Autodesk Inventor part; units mm, degrees
(part 2 of 2)
sketch "Sketch6" plane through (0, 0, 150.495) normal (1, 0, 0) x (0, 0, -1)
  arc A0 (27.7241, 58.674) -> (29.8831, 58.674) centre (28.8036, 58.674) ccw
  line L0 (29.8831, 83.82) -> (29.8831, 58.674)
  line L1 (27.7241, 83.82) -> (27.7241, 58.674)
  line L2 (28.8036, 59.7535) -> (28.8036, 58.674)
  line L3 (28.8036, 83.82) -> (28.8036, 82.7405)
  arc A1 (29.8831, 83.82) -> (27.7241, 83.82) centre (28.8036, 83.82) ccw
  line L4 (28.8036, 55.626) -> (28.8036, 54.5465)
  arc A2 (29.8831, 55.626) -> (27.7241, 55.626) centre (28.8036, 55.626) ccw
  line L5 (27.7241, 55.626) -> (27.7241, 30.48)
  line L6 (29.8831, 55.626) -> (29.8831, 30.48)
  arc A3 (27.7241, 30.48) -> (29.8831, 30.48) centre (28.8036, 30.48) ccw
  line L7 (28.8036, 31.5595) -> (28.8036, 30.48)
  line L8 (28.8036, 27.432) -> (28.8036, 26.3525)
  arc A4 (29.8831, 27.432) -> (27.7241, 27.432) centre (28.8036, 27.432) ccw
  line L9 (29.8831, 27.432) -> (29.8831, 2.286)
  line L10 (27.7241, 27.432) -> (27.7241, 2.286)
  line L11 (28.8036, 3.3655) -> (28.8036, 2.286)
  arc A5 (27.7241, 2.286) -> (29.8831, 2.286) centre (28.8036, 2.286) ccw
  arc A6 (31.8643, 58.674) -> (34.0233, 58.674) centre (32.9438, 58.674) ccw
  line L12 (32.9438, 59.7535) -> (32.9438, 58.674)
  arc A7 (36.0045, 58.674) -> (38.1635, 58.674) centre (37.084, 58.674) ccw
  line L13 (31.8643, 83.82) -> (31.8643, 58.674)
  line L14 (38.1635, 83.82) -> (38.1635, 58.674)
  line L15 (34.0233, 83.82) -> (34.0233, 58.674)
  line L16 (36.0045, 83.82) -> (36.0045, 58.674)
  line L17 (37.084, 59.7535) -> (37.084, 58.674)
  line L18 (32.9438, 83.82) -> (32.9438, 81.8268)
  arc A8 (34.0233, 83.82) -> (31.8643, 83.82) centre (32.9438, 83.82) ccw
  line L19 (37.084, 83.82) -> (37.084, 82.7405)
  arc A9 (38.1635, 83.82) -> (36.0045, 83.82) centre (37.084, 83.82) ccw
  line L20 (32.9438, 55.626) -> (32.9438, 53.2839)
  arc A10 (34.0233, 55.626) -> (31.8643, 55.626) centre (32.9438, 55.626) ccw
  line L21 (37.084, 55.626) -> (37.084, 54.5465)
  arc A11 (38.1635, 55.626) -> (36.0045, 55.626) centre (37.084, 55.626) ccw
  line L22 (31.8643, 55.626) -> (31.8643, 30.48)
  line L23 (32.9438, 31.5595) -> (32.9438, 30.48)
  line L24 (36.0045, 55.626) -> (36.0045, 30.48)
  line L25 (38.1635, 55.626) -> (38.1635, 30.48)
  line L26 (34.0233, 55.626) -> (34.0233, 30.48)
  arc A12 (31.8643, 30.48) -> (34.0233, 30.48) centre (32.9438, 30.48) ccw
  arc A13 (36.0045, 30.48) -> (38.1635, 30.48) centre (37.084, 30.48) ccw
  line L27 (37.084, 31.5595) -> (37.084, 30.48)
  arc A14 (34.0233, 27.432) -> (31.8643, 27.432) centre (32.9438, 27.432) ccw
  line L28 (37.084, 27.432) -> (37.084, 26.3525)
  arc A15 (38.1635, 27.432) -> (36.0045, 27.432) centre (37.084, 27.432) ccw
  line L29 (32.9438, 27.432) -> (32.9438, 26.3525)
  line L30 (38.1635, 27.432) -> (38.1635, 2.286)
  line L31 (36.0045, 27.432) -> (36.0045, 2.286)
  line L32 (34.0233, 27.432) -> (34.0233, 2.286)
  line L33 (31.8643, 27.432) -> (31.8643, 2.286)
  line L34 (37.084, 3.3655) -> (37.084, 2.286)
  line L35 (32.9438, 3.3655) -> (32.9438, 2.286)
  arc A16 (36.0045, 2.286) -> (38.1635, 2.286) centre (37.084, 2.286) ccw
  arc A17 (31.8643, 2.286) -> (34.0233, 2.286) centre (32.9438, 2.286) ccw
  arc A18 (40.1447, 58.674) -> (42.3037, 58.674) centre (41.2242, 58.674) ccw
  line L36 (41.2242, 59.7535) -> (41.2242, 58.674)
  arc A19 (44.2849, 58.674) -> (46.4439, 58.674) centre (45.3644, 58.674) ccw
  line L37 (40.1447, 83.82) -> (40.1447, 58.674)
  line L38 (46.4439, 83.82) -> (46.4439, 58.674)
  line L39 (42.3037, 83.82) -> (42.3037, 58.674)
  line L40 (44.2849, 83.82) -> (44.2849, 58.674)
  line L41 (45.3644, 59.7535) -> (45.3644, 58.674)
  line L42 (41.2242, 83.82) -> (41.2242, 81.8268)
  arc A20 (42.3037, 83.82) -> (40.1447, 83.82) centre (41.2242, 83.82) ccw
  line L43 (45.3644, 83.82) -> (45.3644, 82.7405)
  arc A21 (46.4439, 83.82) -> (44.2849, 83.82) centre (45.3644, 83.82) ccw
  line L44 (41.2242, 55.626) -> (41.2242, 53.2839)
  arc A22 (42.3037, 55.626) -> (40.1447, 55.626) centre (41.2242, 55.626) ccw
  line L45 (45.3644, 55.626) -> (45.3644, 54.5465)
  arc A23 (46.4439, 55.626) -> (44.2849, 55.626) centre (45.3644, 55.626) ccw
  line L46 (40.1447, 55.626) -> (40.1447, 30.48)
  line L47 (41.2242, 31.5595) -> (41.2242, 30.48)
  line L48 (44.2849, 55.626) -> (44.2849, 30.48)
  line L49 (46.4439, 55.626) -> (46.4439, 30.48)
  line L50 (42.3037, 55.626) -> (42.3037, 30.48)
  arc A24 (40.1447, 30.48) -> (42.3037, 30.48) centre (41.2242, 30.48) ccw
  arc A25 (44.2849, 30.48) -> (46.4439, 30.48) centre (45.3644, 30.48) ccw
  line L51 (45.3644, 31.5595) -> (45.3644, 30.48)
  arc A26 (42.3037, 27.432) -> (40.1447, 27.432) centre (41.2242, 27.432) ccw
  line L52 (45.3644, 27.432) -> (45.3644, 26.3525)
  arc A27 (46.4439, 27.432) -> (44.2849, 27.432) centre (45.3644, 27.432) ccw
  line L53 (41.2242, 27.432) -> (41.2242, 26.3525)
  line L54 (46.4439, 27.432) -> (46.4439, 2.286)
  line L55 (44.2849, 27.432) -> (44.2849, 2.286)
  line L56 (42.3037, 27.432) -> (42.3037, 2.286)
  line L57 (40.1447, 27.432) -> (40.1447, 2.286)
  line L58 (45.3644, 3.3655) -> (45.3644, 2.286)
  line L59 (41.2242, 3.3655) -> (41.2242, 2.286)
  arc A28 (44.2849, 2.286) -> (46.4439, 2.286) centre (45.3644, 2.286) ccw
  arc A29 (40.1447, 2.286) -> (42.3037, 2.286) centre (41.2242, 2.286) ccw
  arc A30 (50.5841, 83.82) -> (48.4251, 83.82) centre (49.5046, 83.82) ccw
  line L60 (49.5046, 83.82) -> (49.5046, 81.8268)
  line L61 (53.6448, 83.82) -> (53.6448, 82.7405)
  arc A31 (54.7243, 83.82) -> (52.5653, 83.82) centre (53.6448, 83.82) ccw
  line L62 (48.4251, 83.82) -> (48.4251, 58.674)
  line L63 (49.5046, 59.7535) -> (49.5046, 58.674)
  line L64 (50.5841, 83.82) -> (50.5841, 58.674)
  line L65 (52.5653, 83.82) -> (52.5653, 58.674)
  line L66 (54.7243, 83.82) -> (54.7243, 58.674)
  line L67 (53.6448, 55.626) -> (53.6448, 54.5465)
  line L68 (49.5046, 55.626) -> (49.5046, 53.2839)
  line L69 (54.7243, 55.626) -> (54.7243, 30.48)
  line L70 (53.6448, 31.5595) -> (53.6448, 30.48)
  line L71 (52.5653, 55.626) -> (52.5653, 30.48)
  line L72 (50.5841, 55.626) -> (50.5841, 30.48)
  line L73 (49.5046, 31.5595) -> (49.5046, 30.48)
  line L74 (48.4251, 55.626) -> (48.4251, 30.48)
  arc A32 (50.5841, 55.626) -> (48.4251, 55.626) centre (49.5046, 55.626) ccw
  arc A33 (54.7243, 55.626) -> (52.5653, 55.626) centre (53.6448, 55.626) ccw
  arc A34 (48.4251, 58.674) -> (50.5841, 58.674) centre (49.5046, 58.674) ccw
  arc A35 (52.5653, 58.674) -> (54.7243, 58.674) centre (53.6448, 58.674) ccw
  line L75 (53.6448, 59.7535) -> (53.6448, 58.674)
  arc A36 (52.5653, 30.48) -> (54.7243, 30.48) centre (53.6448, 30.48) ccw
  arc A37 (48.4251, 30.48) -> (50.5841, 30.48) centre (49.5046, 30.48) ccw
  arc A38 (54.7243, 27.432) -> (52.5653, 27.432) centre (53.6448, 27.432) ccw
  arc A39 (50.5841, 27.432) -> (48.4251, 27.432) centre (49.5046, 27.432) ccw
  line L76 (49.5046, 27.432) -> (49.5046, 26.3525)
  line L77 (53.6448, 27.432) -> (53.6448, 26.3525)
  line L78 (54.7243, 27.432) -> (54.7243, 2.286)
  line L79 (52.5653, 27.432) -> (52.5653, 2.286)
  line L80 (50.5841, 27.432) -> (50.5841, 2.286)
  line L81 (48.4251, 27.432) -> (48.4251, 2.286)
  line L82 (53.6448, 3.3655) -> (53.6448, 2.286)
  line L83 (49.5046, 3.3655) -> (49.5046, 2.286)
  arc A40 (52.5653, 2.286) -> (54.7243, 2.286) centre (53.6448, 2.286) ccw
  arc A41 (48.4251, 2.286) -> (50.5841, 2.286) centre (49.5046, 2.286) ccw
  arc A42 (58.8645, 83.82) -> (56.7055, 83.82) centre (57.785, 83.82) ccw
  line L84 (57.785, 83.82) -> (57.785, 81.8268)
  line L85 (61.9252, 83.82) -> (61.9252, 82.7405)
  arc A43 (63.0047, 83.82) -> (60.8457, 83.82) centre (61.9252, 83.82) ccw
  line L86 (56.7055, 83.82) -> (56.7055, 58.674)
  line L87 (57.785, 59.7535) -> (57.785, 58.674)
  line L88 (58.8645, 83.82) -> (58.8645, 58.674)
  line L89 (60.8457, 83.82) -> (60.8457, 58.674)
  line L90 (63.0047, 83.82) -> (63.0047, 58.674)
  line L91 (61.9252, 55.626) -> (61.9252, 54.5465)
  line L92 (57.785, 55.626) -> (57.785, 53.2839)
  line L93 (63.0047, 55.626) -> (63.0047, 30.48)
  line L94 (61.9252, 31.5595) -> (61.9252, 30.48)
  line L95 (60.8457, 55.626) -> (60.8457, 30.48)
  line L96 (58.8645, 55.626) -> (58.8645, 30.48)
  line L97 (57.785, 31.5595) -> (57.785, 30.48)
  line L98 (56.7055, 55.626) -> (56.7055, 30.48)
  arc A44 (58.8645, 55.626) -> (56.7055, 55.626) centre (57.785, 55.626) ccw
  arc A45 (63.0047, 55.626) -> (60.8457, 55.626) centre (61.9252, 55.626) ccw
  arc A46 (56.7055, 58.674) -> (58.8645, 58.674) centre (57.785, 58.674) ccw
  arc A47 (60.8457, 58.674) -> (63.0047, 58.674) centre (61.9252, 58.674) ccw
  line L99 (61.9252, 59.7535) -> (61.9252, 58.674)
  arc A48 (60.8457, 30.48) -> (63.0047, 30.48) centre (61.9252, 30.48) ccw
  arc A49 (56.7055, 30.48) -> (58.8645, 30.48) centre (57.785, 30.48) ccw
  arc A50 (63.0047, 27.432) -> (60.8457, 27.432) centre (61.9252, 27.432) ccw
  arc A51 (58.8645, 27.432) -> (56.7055, 27.432) centre (57.785, 27.432) ccw
  line L100 (57.785, 27.432) -> (57.785, 26.3525)
  line L101 (61.9252, 27.432) -> (61.9252, 26.3525)
  line L102 (63.0047, 27.432) -> (63.0047, 2.286)
  line L103 (60.8457, 27.432) -> (60.8457, 2.286)
  line L104 (58.8645, 27.432) -> (58.8645, 2.286)
  line L105 (56.7055, 27.432) -> (56.7055, 2.286)
  line L106 (61.9252, 3.3655) -> (61.9252, 2.286)
  line L107 (57.785, 3.3655) -> (57.785, 2.286)
  arc A52 (60.8457, 2.286) -> (63.0047, 2.286) centre (61.9252, 2.286) ccw
  arc A53 (56.7055, 2.286) -> (58.8645, 2.286) centre (57.785, 2.286) ccw
  arc A54 (67.1449, 83.82) -> (64.9859, 83.82) centre (66.0654, 83.82) ccw
  line L108 (66.0654, 83.82) -> (66.0654, 81.8268)
  line L109 (70.2056, 83.82) -> (70.2056, 82.7405)
  arc A55 (71.2851, 83.82) -> (69.1261, 83.82) centre (70.2056, 83.82) ccw
  line L110 (64.9859, 83.82) -> (64.9859, 58.674)
  line L111 (66.0654, 59.7535) -> (66.0654, 58.674)
  line L112 (67.1449, 83.82) -> (67.1449, 58.674)
  line L113 (69.1261, 83.82) -> (69.1261, 58.674)
  line L114 (71.2851, 83.82) -> (71.2851, 58.674)
  line L115 (70.2056, 55.626) -> (70.2056, 54.5465)
  line L116 (66.0654, 55.626) -> (66.0654, 53.2839)
  line L117 (71.2851, 55.626) -> (71.2851, 30.48)
  line L118 (70.2056, 31.5595) -> (70.2056, 30.48)
  line L119 (69.1261, 55.626) -> (69.1261, 30.48)
  line L120 (67.1449, 55.626) -> (67.1449, 30.48)
  line L121 (66.0654, 31.5595) -> (66.0654, 30.48)
  line L122 (64.9859, 55.626) -> (64.9859, 30.48)
  arc A56 (67.1449, 55.626) -> (64.9859, 55.626) centre (66.0654, 55.626) ccw
  arc A57 (71.2851, 55.626) -> (69.1261, 55.626) centre (70.2056, 55.626) ccw
  arc A58 (64.9859, 58.674) -> (67.1449, 58.674) centre (66.0654, 58.674) ccw
  arc A59 (69.1261, 58.674) -> (71.2851, 58.674) centre (70.2056, 58.674) ccw
  line L123 (70.2056, 59.7535) -> (70.2056, 58.674)
  arc A60 (69.1261, 30.48) -> (71.2851, 30.48) centre (70.2056, 30.48) ccw
  arc A61 (64.9859, 30.48) -> (67.1449, 30.48) centre (66.0654, 30.48) ccw
  arc A62 (71.2851, 27.432) -> (69.1261, 27.432) centre (70.2056, 27.432) ccw
  arc A63 (67.1449, 27.432) -> (64.9859, 27.432) centre (66.0654, 27.432) ccw
  line L124 (66.0654, 27.432) -> (66.0654, 26.3525)
  line L125 (70.2056, 27.432) -> (70.2056, 26.3525)
  line L126 (71.2851, 27.432) -> (71.2851, 2.286)
  line L127 (69.1261, 27.432) -> (69.1261, 2.286)
  line L128 (67.1449, 27.432) -> (67.1449, 2.286)
  line L129 (64.9859, 27.432) -> (64.9859, 2.286)
  line L130 (70.2056, 3.3655) -> (70.2056, 2.286)
  line L131 (66.0654, 3.3655) -> (66.0654, 2.286)
  arc A64 (69.1261, 2.286) -> (71.2851, 2.286) centre (70.2056, 2.286) ccw
  arc A65 (64.9859, 2.286) -> (67.1449, 2.286) centre (66.0654, 2.286) ccw
  arc A66 (73.2663, 58.674) -> (75.4253, 58.674) centre (74.3458, 58.674) ccw
  line L132 (74.3458, 59.7535) -> (74.3458, 58.674)
  arc A67 (77.4065, 58.674) -> (79.5655, 58.674) centre (78.486, 58.674) ccw
  line L133 (73.2663, 83.82) -> (73.2663, 58.674)
  line L134 (79.5655, 83.82) -> (79.5655, 58.674)
  line L135 (75.4253, 83.82) -> (75.4253, 58.674)
  line L136 (77.4065, 83.82) -> (77.4065, 58.674)
  line L137 (78.486, 59.7535) -> (78.486, 58.674)
  line L138 (74.3458, 83.82) -> (74.3458, 81.8268)
  arc A68 (75.4253, 83.82) -> (73.2663, 83.82) centre (74.3458, 83.82) ccw
  line L139 (78.486, 83.82) -> (78.486, 82.7405)
  arc A69 (79.5655, 83.82) -> (77.4065, 83.82) centre (78.486, 83.82) ccw
  line L140 (74.3458, 55.626) -> (74.3458, 53.2839)
  arc A70 (75.4253, 55.626) -> (73.2663, 55.626) centre (74.3458, 55.626) ccw
  line L141 (78.486, 55.626) -> (78.486, 54.5465)
  arc A71 (79.5655, 55.626) -> (77.4065, 55.626) centre (78.486, 55.626) ccw
  line L142 (73.2663, 55.626) -> (73.2663, 30.48)
  line L143 (74.3458, 31.5595) -> (74.3458, 30.48)
  line L144 (77.4065, 55.626) -> (77.4065, 30.48)
  line L145 (79.5655, 55.626) -> (79.5655, 30.48)
  line L146 (75.4253, 55.626) -> (75.4253, 30.48)
  arc A72 (73.2663, 30.48) -> (75.4253, 30.48) centre (74.3458, 30.48) ccw
  arc A73 (77.4065, 30.48) -> (79.5655, 30.48) centre (78.486, 30.48) ccw
  line L147 (78.486, 31.5595) -> (78.486, 30.48)
  arc A74 (75.4253, 27.432) -> (73.2663, 27.432) centre (74.3458, 27.432) ccw
  line L148 (78.486, 27.432) -> (78.486, 26.3525)
  arc A75 (79.5655, 27.432) -> (77.4065, 27.432) centre (78.486, 27.432) ccw
  line L149 (74.3458, 27.432) -> (74.3458, 26.3525)
  line L150 (79.5655, 27.432) -> (79.5655, 2.286)
  line L151 (77.4065, 27.432) -> (77.4065, 2.286)
  line L152 (75.4253, 27.432) -> (75.4253, 2.286)
  line L153 (73.2663, 27.432) -> (73.2663, 2.286)
  line L154 (78.486, 3.3655) -> (78.486, 2.286)
  line L155 (74.3458, 3.3655) -> (74.3458, 2.286)
  arc A76 (77.4065, 2.286) -> (79.5655, 2.286) centre (78.486, 2.286) ccw
  arc A77 (73.2663, 2.286) -> (75.4253, 2.286) centre (74.3458, 2.286) ccw
  arc A78 (83.7057, 83.82) -> (81.5467, 83.82) centre (82.6262, 83.82) ccw
  line L156 (82.6262, 83.82) -> (82.6262, 81.8268)
  line L157 (86.7664, 83.82) -> (86.7664, 82.7405)
  arc A79 (87.8459, 83.82) -> (85.6869, 83.82) centre (86.7664, 83.82) ccw
  line L158 (81.5467, 83.82) -> (81.5467, 58.674)
  line L159 (82.6262, 59.7535) -> (82.6262, 58.674)
  line L160 (83.7057, 83.82) -> (83.7057, 58.674)
  line L161 (85.6869, 83.82) -> (85.6869, 58.674)
  line L162 (87.8459, 83.82) -> (87.8459, 58.674)
  line L163 (86.7664, 55.626) -> (86.7664, 54.5465)
  line L164 (82.6262, 55.626) -> (82.6262, 53.2839)
  line L165 (87.8459, 55.626) -> (87.8459, 30.48)
  line L166 (86.7664, 31.5595) -> (86.7664, 30.48)
  line L167 (85.6869, 55.626) -> (85.6869, 30.48)
  line L168 (83.7057, 55.626) -> (83.7057, 30.48)
  line L169 (82.6262, 31.5595) -> (82.6262, 30.48)
  line L170 (81.5467, 55.626) -> (81.5467, 30.48)
  arc A80 (83.7057, 55.626) -> (81.5467, 55.626) centre (82.6262, 55.626) ccw
  arc A81 (87.8459, 55.626) -> (85.6869, 55.626) centre (86.7664, 55.626) ccw
  arc A82 (81.5467, 58.674) -> (83.7057, 58.674) centre (82.6262, 58.674) ccw
  arc A83 (85.6869, 58.674) -> (87.8459, 58.674) centre (86.7664, 58.674) ccw
  line L171 (86.7664, 59.7535) -> (86.7664, 58.674)
  arc A84 (85.6869, 30.48) -> (87.8459, 30.48) centre (86.7664, 30.48) ccw
  arc A85 (81.5467, 30.48) -> (83.7057, 30.48) centre (82.6262, 30.48) ccw
  arc A86 (87.8459, 27.432) -> (85.6869, 27.432) centre (86.7664, 27.432) ccw
  arc A87 (83.7057, 27.432) -> (81.5467, 27.432) centre (82.6262, 27.432) ccw
  line L172 (82.6262, 27.432) -> (82.6262, 26.3525)
  line L173 (86.7664, 27.432) -> (86.7664, 26.3525)
  line L174 (87.8459, 27.432) -> (87.8459, 2.286)
  line L175 (85.6869, 27.432) -> (85.6869, 2.286)
  line L176 (83.7057, 27.432) -> (83.7057, 2.286)
  line L177 (81.5467, 27.432) -> (81.5467, 2.286)
  line L178 (86.7664, 3.3655) -> (86.7664, 2.286)
  line L179 (82.6262, 3.3655) -> (82.6262, 2.286)
  arc A88 (85.6869, 2.286) -> (87.8459, 2.286) centre (86.7664, 2.286) ccw
  arc A89 (81.5467, 2.286) -> (83.7057, 2.286) centre (82.6262, 2.286) ccw
  arc A90 (91.9861, 83.82) -> (89.8271, 83.82) centre (90.9066, 83.82) ccw
  line L180 (90.9066, 83.82) -> (90.9066, 81.8268)
  line L181 (95.0468, 83.82) -> (95.0468, 82.7405)
  arc A91 (96.1263, 83.82) -> (93.9673, 83.82) centre (95.0468, 83.82) ccw
  line L182 (89.8271, 83.82) -> (89.8271, 58.674)
  line L183 (90.9066, 59.7535) -> (90.9066, 58.674)
  line L184 (91.9861, 83.82) -> (91.9861, 58.674)
  line L185 (93.9673, 83.82) -> (93.9673, 58.674)
  line L186 (96.1263, 83.82) -> (96.1263, 58.674)
  line L187 (95.0468, 55.626) -> (95.0468, 54.5465)
  line L188 (90.9066, 55.626) -> (90.9066, 53.2839)
  line L189 (96.1263, 55.626) -> (96.1263, 30.48)
  line L190 (95.0468, 31.5595) -> (95.0468, 30.48)
  line L191 (93.9673, 55.626) -> (93.9673, 30.48)
  line L192 (91.9861, 55.626) -> (91.9861, 30.48)
  line L193 (90.9066, 31.5595) -> (90.9066, 30.48)
  line L194 (89.8271, 55.626) -> (89.8271, 30.48)
  arc A92 (91.9861, 55.626) -> (89.8271, 55.626) centre (90.9066, 55.626) ccw
  arc A93 (96.1263, 55.626) -> (93.9673, 55.626) centre (95.0468, 55.626) ccw
  arc A94 (89.8271, 58.674) -> (91.9861, 58.674) centre (90.9066, 58.674) ccw
  arc A95 (93.9673, 58.674) -> (96.1263, 58.674) centre (95.0468, 58.674) ccw
  line L195 (95.0468, 59.7535) -> (95.0468, 58.674)
  arc A96 (93.9673, 30.48) -> (96.1263, 30.48) centre (95.0468, 30.48) ccw
  arc A97 (89.8271, 30.48) -> (91.9861, 30.48) centre (90.9066, 30.48) ccw
  arc A98 (96.1263, 27.432) -> (93.9673, 27.432) centre (95.0468, 27.432) ccw
  arc A99 (91.9861, 27.432) -> (89.8271, 27.432) centre (90.9066, 27.432) ccw
  line L196 (90.9066, 27.432) -> (90.9066, 26.3525)
  line L197 (95.0468, 27.432) -> (95.0468, 26.3525)
  line L198 (96.1263, 27.432) -> (96.1263, 2.286)
  line L199 (93.9673, 27.432) -> (93.9673, 2.286)
  line L200 (91.9861, 27.432) -> (91.9861, 2.286)
  line L201 (89.8271, 27.432) -> (89.8271, 2.286)
  line L202 (95.0468, 3.3655) -> (95.0468, 2.286)
  line L203 (90.9066, 3.3655) -> (90.9066, 2.286)
  arc A100 (93.9673, 2.286) -> (96.1263, 2.286) centre (95.0468, 2.286) ccw
  arc A101 (89.8271, 2.286) -> (91.9861, 2.286) centre (90.9066, 2.286) ccw
  arc A102 (100.2665, 83.82) -> (98.1075, 83.82) centre (99.187, 83.82) ccw
  line L204 (99.187, 83.82) -> (99.187, 81.8268)
  line L205 (103.3272, 83.82) -> (103.3272, 82.7405)
  arc A103 (104.4067, 83.82) -> (102.2477, 83.82) centre (103.3272, 83.82) ccw
  line L206 (98.1075, 83.82) -> (98.1075, 58.674)
  line L207 (99.187, 59.7535) -> (99.187, 58.674)
  line L208 (100.2665, 83.82) -> (100.2665, 58.674)
  line L209 (102.2477, 83.82) -> (102.2477, 58.674)
  line L210 (104.4067, 83.82) -> (104.4067, 58.674)
  line L211 (103.3272, 55.626) -> (103.3272, 54.5465)
  line L212 (99.187, 55.626) -> (99.187, 53.2839)
  line L213 (104.4067, 55.626) -> (104.4067, 30.48)
  line L214 (103.3272, 31.5595) -> (103.3272, 30.48)
  line L215 (102.2477, 55.626) -> (102.2477, 30.48)
  line L216 (100.2665, 55.626) -> (100.2665, 30.48)
  line L217 (99.187, 31.5595) -> (99.187, 30.48)
  line L218 (98.1075, 55.626) -> (98.1075, 30.48)
  arc A104 (100.2665, 55.626) -> (98.1075, 55.626) centre (99.187, 55.626) ccw
  arc A105 (104.4067, 55.626) -> (102.2477, 55.626) centre (103.3272, 55.626) ccw
  arc A106 (98.1075, 58.674) -> (100.2665, 58.674) centre (99.187, 58.674) ccw
  arc A107 (102.2477, 58.674) -> (104.4067, 58.674) centre (103.3272, 58.674) ccw
  line L219 (103.3272, 59.7535) -> (103.3272, 58.674)
  arc A108 (102.2477, 30.48) -> (104.4067, 30.48) centre (103.3272, 30.48) ccw
  arc A109 (98.1075, 30.48) -> (100.2665, 30.48) centre (99.187, 30.48) ccw
  arc A110 (104.4067, 27.432) -> (102.2477, 27.432) centre (103.3272, 27.432) ccw
  arc A111 (100.2665, 27.432) -> (98.1075, 27.432) centre (99.187, 27.432) ccw
  line L220 (99.187, 27.432) -> (99.187, 26.3525)
  line L221 (103.3272, 27.432) -> (103.3272, 26.3525)
  line L222 (104.4067, 27.432) -> (104.4067, 2.286)
  line L223 (102.2477, 27.432) -> (102.2477, 2.286)
  line L224 (100.2665, 27.432) -> (100.2665, 2.286)
  line L225 (98.1075, 27.432) -> (98.1075, 2.286)
  line L226 (103.3272, 3.3655) -> (103.3272, 2.286)
  line L227 (99.187, 3.3655) -> (99.187, 2.286)
  arc A112 (102.2477, 2.286) -> (104.4067, 2.286) centre (103.3272, 2.286) ccw
  arc A113 (98.1075, 2.286) -> (100.2665, 2.286) centre (99.187, 2.286) ccw
  arc A114 (106.3879, 58.674) -> (108.5469, 58.674) centre (107.4674, 58.674) ccw
  arc A115 (110.5281, 58.674) -> (112.6871, 58.674) centre (111.6076, 58.674) ccw
  line L228 (111.6076, 59.7535) -> (111.6076, 58.674)
  arc A116 (112.6871, 55.626) -> (110.5281, 55.626) centre (111.6076, 55.626) ccw
  arc A117 (108.5469, 55.626) -> (106.3879, 55.626) centre (107.4674, 55.626) ccw
  line L229 (115.7478, 59.7535) -> (115.7478, 58.674)
  arc A118 (116.8273, 55.626) -> (114.6683, 55.626) centre (115.7478, 55.626) ccw
  arc A119 (120.9675, 55.626) -> (118.8085, 55.626) centre (119.888, 55.626) ccw
  arc A120 (114.6683, 58.674) -> (116.8273, 58.674) centre (115.7478, 58.674) ccw
  arc A121 (118.8085, 58.674) -> (120.9675, 58.674) centre (119.888, 58.674) ccw
  line L230 (119.888, 59.7535) -> (119.888, 58.674)
  line L231 (124.0282, 59.7535) -> (124.0282, 58.674)
  arc A122 (125.1077, 55.626) -> (122.9487, 55.626) centre (124.0282, 55.626) ccw
  arc A123 (122.9487, 58.674) -> (125.1077, 58.674) centre (124.0282, 58.674) ccw
  line L232 (107.4674, 83.82) -> (107.4674, 81.8268)
  arc A124 (108.5469, 83.82) -> (106.3879, 83.82) centre (107.4674, 83.82) ccw
  arc A125 (116.8273, 83.82) -> (114.6683, 83.82) centre (115.7478, 83.82) ccw
  arc A126 (112.6871, 83.82) -> (110.5281, 83.82) centre (111.6076, 83.82) ccw
  line L233 (111.6076, 83.82) -> (111.6076, 82.7405)
  line L234 (119.888, 83.82) -> (119.888, 82.7405)
  line L235 (124.0282, 83.82) -> (124.0282, 81.8268)
  arc A127 (125.1077, 83.82) -> (122.9487, 83.82) centre (124.0282, 83.82) ccw
  arc A128 (120.9675, 83.82) -> (118.8085, 83.82) centre (119.888, 83.82) ccw
  line L236 (120.9675, 83.82) -> (120.9675, 58.674)
  line L237 (122.9487, 83.82) -> (122.9487, 58.674)
  line L238 (125.1077, 83.82) -> (125.1077, 58.674)
  line L239 (119.888, 3.3655) -> (119.888, 2.286)
  arc A129 (122.9487, 2.286) -> (125.1077, 2.286) centre (124.0282, 2.286) ccw
  arc A130 (118.8085, 2.286) -> (120.9675, 2.286) centre (119.888, 2.286) ccw
  line L240 (115.7478, 3.3655) -> (115.7478, 2.286)
  line L241 (124.0282, 3.3655) -> (124.0282, 2.286)
  line L242 (125.1077, 27.432) -> (125.1077, 2.286)
  line L243 (122.9487, 27.432) -> (122.9487, 2.286)
  line L244 (120.9675, 27.432) -> (120.9675, 2.286)
  line L245 (118.8085, 27.432) -> (118.8085, 2.286)
  line L246 (114.6683, 27.432) -> (114.6683, 2.286)
  line L247 (112.6871, 27.432) -> (112.6871, 2.286)
  line L248 (110.5281, 27.432) -> (110.5281, 2.286)
  line L249 (108.5469, 27.432) -> (108.5469, 2.286)
  line L250 (106.3879, 27.432) -> (106.3879, 2.286)
  line L251 (116.8273, 27.432) -> (116.8273, 2.286)
  line L252 (111.6076, 27.432) -> (111.6076, 26.3525)
  line L253 (107.4674, 27.432) -> (107.4674, 26.3525)
  line L254 (111.6076, 3.3655) -> (111.6076, 2.286)
  line L255 (107.4674, 3.3655) -> (107.4674, 2.286)
  arc A131 (110.5281, 2.286) -> (112.6871, 2.286) centre (111.6076, 2.286) ccw
  arc A132 (106.3879, 2.286) -> (108.5469, 2.286) centre (107.4674, 2.286) ccw
  arc A133 (114.6683, 2.286) -> (116.8273, 2.286) centre (115.7478, 2.286) ccw
  line L256 (115.7478, 83.82) -> (115.7478, 81.8268)
  line L257 (116.8273, 83.82) -> (116.8273, 58.674)
  line L258 (114.6683, 83.82) -> (114.6683, 58.674)
  line L259 (112.6871, 83.82) -> (112.6871, 58.674)
  line L260 (108.5469, 83.82) -> (108.5469, 58.674)
  line L261 (107.4674, 59.7535) -> (107.4674, 58.674)
  line L262 (106.3879, 83.82) -> (106.3879, 58.674)
  line L263 (110.5281, 83.82) -> (110.5281, 58.674)
  line L264 (107.4674, 55.626) -> (107.4674, 53.2839)
  line L265 (111.6076, 55.626) -> (111.6076, 54.5465)
  line L266 (115.7478, 55.626) -> (115.7478, 53.2839)
  line L267 (119.888, 55.626) -> (119.888, 54.5465)
  line L268 (124.0282, 55.626) -> (124.0282, 53.2839)
  line L269 (106.3879, 55.626) -> (106.3879, 30.48)
  line L270 (108.5469, 55.626) -> (108.5469, 30.48)
  line L271 (110.5281, 55.626) -> (110.5281, 30.48)
  line L272 (112.6871, 55.626) -> (112.6871, 30.48)
  line L273 (114.6683, 55.626) -> (114.6683, 30.48)
  line L274 (118.8085, 55.626) -> (118.8085, 30.48)
  line L275 (120.9675, 55.626) -> (120.9675, 30.48)
  line L276 (122.9487, 55.626) -> (122.9487, 30.48)
  line L277 (125.1077, 55.626) -> (125.1077, 30.48)
  line L278 (116.8273, 55.626) -> (116.8273, 30.48)
  line L279 (118.8085, 83.82) -> (118.8085, 58.674)
  line L280 (124.0282, 31.5595) -> (124.0282, 30.48)
  line L281 (119.888, 31.5595) -> (119.888, 30.48)
  line L282 (115.7478, 31.5595) -> (115.7478, 30.48)
  arc A134 (110.5281, 30.48) -> (112.6871, 30.48) centre (111.6076, 30.48) ccw
  line L283 (111.6076, 31.5595) -> (111.6076, 30.48)
  arc A135 (112.6871, 27.432) -> (110.5281, 27.432) centre (111.6076, 27.432) ccw
  line L284 (107.4674, 31.5595) -> (107.4674, 30.48)
  arc A136 (106.3879, 30.48) -> (108.5469, 30.48) centre (107.4674, 30.48) ccw
  arc A137 (108.5469, 27.432) -> (106.3879, 27.432) centre (107.4674, 27.432) ccw
  arc A138 (118.8085, 30.48) -> (120.9675, 30.48) centre (119.888, 30.48) ccw
  arc A139 (114.6683, 30.48) -> (116.8273, 30.48) centre (115.7478, 30.48) ccw
  line L285 (119.888, 27.432) -> (119.888, 26.3525)
  line L286 (115.7478, 27.432) -> (115.7478, 26.3525)
  arc A140 (120.9675, 27.432) -> (118.8085, 27.432) centre (119.888, 27.432) ccw
  arc A141 (116.8273, 27.432) -> (114.6683, 27.432) centre (115.7478, 27.432) ccw
  line L287 (124.0282, 27.432) -> (124.0282, 26.3525)
  arc A142 (125.1077, 27.432) -> (122.9487, 27.432) centre (124.0282, 27.432) ccw
  arc A143 (122.9487, 30.48) -> (125.1077, 30.48) centre (124.0282, 30.48) ccw
  dimension "d223" = 25.146
  dimension "d226" = 25.146
  dimension "d230" = 25.146
  dimension "d234" = 25.146
  dimension "d235" = 25.146
  dimension "d236" = 4.1402
  dimension "d237" = 25.146
  dimension "d238" = 25.146
  dimension "d239" = 4.1402
  dimension "d240" = 0
  dimension "d241" = 25.146
  dimension "d242" = 25.146
  dimension "d243" = 4.1402
  dimension "d244" = 3.048
  dimension "d245" = 3.048
  dimension "d248" = 4.1402
  dimension "d249" = 25.146
  dimension "d250" = 25.146
  dimension "d251" = 4.1402
  dimension "d252" = 25.146
  dimension "d253" = 25.146
  dimension "d254" = 4.1402
  dimension "d255" = 0
  dimension "d256" = 25.146
  dimension "d257" = 25.146
  dimension "d258" = 4.1402
  dimension "d259" = 3.048
  dimension "d260" = 3.048
  dimension "d261" = 25.146
  dimension "d262" = 25.146
  dimension "d263" = 4.1402
  dimension "d264" = 25.146
  dimension "d265" = 25.146
  dimension "d266" = 4.1402
  dimension "d267" = 0
  dimension "d268" = 25.146
  dimension "d269" = 25.146
  dimension "d270" = 4.1402
  dimension "d271" = 3.048
  dimension "d272" = 3.048
  dimension "d273" = 25.146
  dimension "d274" = 25.146
  dimension "d275" = 4.1402
  dimension "d276" = 25.146
  dimension "d277" = 25.146
  dimension "d278" = 4.1402
  dimension "d279" = 0
  dimension "d280" = 25.146
  dimension "d281" = 25.146
  dimension "d282" = 4.1402
  dimension "d283" = 3.048
  dimension "d284" = 3.048
  dimension "d285" = 25.146
  dimension "d286" = 25.146
  dimension "d287" = 4.1402
  dimension "d288" = 25.146
  dimension "d289" = 25.146
  dimension "d290" = 4.1402
  dimension "d291" = 0
  dimension "d292" = 25.146
  dimension "d293" = 25.146
  dimension "d294" = 4.1402
  dimension "d295" = 3.048
  dimension "d296" = 3.048
  constraints: 576 end point, 288 point on circle, 216 parallel, 144 centre point, 108 coincident, 72 tangent
  measures "d223" distance of L3.start L2.end
  measures "d226" distance of L4.start L7.end
  measures "d230" distance of L8.start L11.end
  measures "d234" distance of L18.start L12.end
  measures "d235" distance of L19.start L17.end
  measures "d236" distance between parallel lines of L17 L12
  measures "d237" distance of L20.start L23.end
  measures "d238" distance of L21.start L27.end
  measures "d239" distance between parallel lines of L27 L23
  measures "d240" distance between parallel lines of L12 L20
  measures "d241" distance of L29.start L35.end
  measures "d242" distance of L28.start L34.end
  measures "d243" distance between parallel lines of L34 L35
  measures "d244" distance of L23.end L29.start
  measures "d245" distance of A6.centre L20.start
  measures "d248" distance between parallel lines of L3 L18
  measures "d249" distance of L42.start L36.end
  measures "d250" distance of L43.start L41.end
  measures "d251" distance between parallel lines of L41 L36
  measures "d252" distance of L44.start L47.end
  measures "d253" distance of L45.start L51.end
  measures "d254" distance between parallel lines of L51 L47
  measures "d255" distance between parallel lines of L36 L44
  measures "d256" distance of L53.start L59.end
  measures "d257" distance of L52.start L58.end
  measures "d258" distance between parallel lines of L58 L59
  measures "d259" distance of L47.end L53.start
  measures "d260" distance of A18.centre L44.start
  measures "d261" distance of L60.start L63.end
  measures "d262" distance of L61.start L75.end
  measures "d263" distance between parallel lines of L75 L63
  measures "d264" distance of L68.start L73.end
  measures "d265" distance of L67.start L70.end
  measures "d266" distance between parallel lines of L70 L73
  measures "d267" distance between parallel lines of L63 L68
  measures "d268" distance of L76.start L83.end
  measures "d269" distance of L77.start L82.end
  measures "d270" distance between parallel lines of L82 L83
  measures "d271" distance of L73.end L76.start
  measures "d272" distance of A34.centre L68.start
  measures "d273" distance of L84.start L87.end
  measures "d274" distance of L85.start L99.end
  measures "d275" distance between parallel lines of L99 L87
  measures "d276" distance of L92.start L97.end
  measures "d277" distance of L91.start L94.end
  measures "d278" distance between parallel lines of L94 L97
  measures "d279" distance between parallel lines of L87 L92
  measures "d280" distance of L100.start L107.end
  measures "d281" distance of L101.start L106.end
  measures "d282" distance between parallel lines of L106 L107
  measures "d283" distance of L97.end L100.start
  measures "d284" distance of A46.centre L92.start
  measures "d285" distance of L108.start L111.end
  measures "d286" distance of L109.start L123.end
  measures "d287" distance between parallel lines of L123 L111
  measures "d288" distance of L116.start L121.end
  measures "d289" distance of L115.start L118.end
  measures "d290" distance between parallel lines of L118 L121
  measures "d291" distance between parallel lines of L111 L116
  measures "d292" distance of L124.start L131.end
  measures "d293" distance of L125.start L130.end
  measures "d294" distance between parallel lines of L130 L131
  measures "d295" distance of L121.end L124.start
  measures "d296" distance of A58.centre L116.start
extrude "Extrusion5" cut sketch "Sketch6" against normal blind 50.8
sketch "Sketch8" plane through (-141.224, 0, 0) normal (-1, 0, 0) x (0, 0, 1)
  circle A0 centre (46.7921, 42.926) radius 40.8714
  circle A1 centre (46.7921, 42.926) radius 36.5016
  circle A2 centre (46.7921, 42.926) radius 34.1821
  circle A3 centre (46.7921, 42.926) radius 29.2524
  circle A4 centre (46.7921, 42.926) radius 27.2128
  circle A5 centre (46.7921, 42.926) radius 21.9649
  circle A6 centre (46.7921, 42.926) radius 19.7247
  circle A7 centre (46.7921, 42.926) radius 14.2135
  circle A8 centre (46.7921, 48.8564) radius 1.789
  line L0 (49.1955, 79.3483) -> (49.1955, 83.7266)
  line L1 (44.3888, 79.3483) -> (44.3888, 83.7266)
  line L2 (49.1955, 77.0236) -> (49.1955, 72.0795)
  line L3 (44.3888, 77.0236) -> (44.3888, 72.0795)
  line L4 (44.3888, 70.0325) -> (44.3888, 64.759)
  line L5 (49.1955, 70.0325) -> (49.1955, 64.759)
  line L6 (44.3888, 62.5037) -> (44.3888, 56.9349)
  line L7 (49.1955, 62.5037) -> (49.1955, 56.9349)
  circle A9 centre (46.7921, 48.8564) radius 3.7241
  circle A10 centre (46.7921, 42.926) radius 40.8714
  circle A11 centre (46.7921, 42.926) radius 36.5016
  circle A12 centre (46.7921, 42.926) radius 34.1821
  circle A13 centre (46.7921, 42.926) radius 29.2524
  circle A14 centre (46.7921, 42.926) radius 27.2128
  circle A15 centre (46.7921, 42.926) radius 21.9649
  circle A16 centre (46.7921, 42.926) radius 19.7247
  circle A17 centre (46.7921, 42.926) radius 14.2135
  line L8 (16.4511, 63.2185) -> (12.6594, 65.4077)
  line L9 (14.0478, 59.0558) -> (10.2561, 61.245)
  line L10 (18.4645, 62.0561) -> (22.7461, 59.5841)
  line L11 (16.0611, 57.8934) -> (20.3428, 55.4214)
  line L12 (22.1156, 54.3979) -> (26.6826, 51.7612)
  line L13 (24.5189, 58.5606) -> (29.0859, 55.9238)
  line L14 (28.6357, 50.6335) -> (33.4584, 47.8491)
  line L15 (31.039, 54.7962) -> (35.8618, 52.0118)
  circle A18 centre (46.7921, 42.926) radius 40.8714
  circle A19 centre (46.7921, 42.926) radius 36.5016
  circle A20 centre (46.7921, 42.926) radius 34.1821
  circle A21 centre (46.7921, 42.926) radius 29.2524
  circle A22 centre (46.7921, 42.926) radius 27.2128
  circle A23 centre (46.7921, 42.926) radius 21.9649
  circle A24 centre (46.7921, 42.926) radius 19.7247
  circle A25 centre (46.7921, 42.926) radius 14.2135
  line L16 (14.0478, 26.7962) -> (10.2561, 24.607)
  line L17 (16.4511, 22.6335) -> (12.6594, 20.4443)
  line L18 (16.0611, 27.9586) -> (20.3428, 30.4306)
  line L19 (18.4645, 23.7959) -> (22.7461, 26.2679)
  line L20 (24.5189, 27.2914) -> (29.0859, 29.9282)
  line L21 (22.1156, 31.4541) -> (26.6826, 34.0908)
  line L22 (31.039, 31.0558) -> (35.8618, 33.8402)
  line L23 (28.6357, 35.2185) -> (33.4584, 38.0029)
  circle A26 centre (46.7921, 42.926) radius 40.8714
  circle A27 centre (46.7921, 42.926) radius 36.5016
  circle A28 centre (46.7921, 42.926) radius 34.1821
  circle A29 centre (46.7921, 42.926) radius 29.2524
  circle A30 centre (46.7921, 42.926) radius 27.2128
  circle A31 centre (46.7921, 42.926) radius 21.9649
  circle A32 centre (46.7921, 42.926) radius 19.7247
  circle A33 centre (46.7921, 42.926) radius 14.2135
  line L24 (44.3888, 6.5037) -> (44.3888, 2.1254)
  line L25 (49.1955, 6.5037) -> (49.1955, 2.1254)
  line L26 (44.3888, 8.8284) -> (44.3888, 13.7725)
  line L27 (49.1955, 8.8284) -> (49.1955, 13.7725)
  line L28 (49.1955, 15.8195) -> (49.1955, 21.093)
  line L29 (44.3888, 15.8195) -> (44.3888, 21.093)
  line L30 (49.1955, 23.3483) -> (49.1955, 28.9171)
  line L31 (44.3888, 23.3483) -> (44.3888, 28.9171)
  circle A34 centre (46.7921, 42.926) radius 40.8714
  circle A35 centre (46.7921, 42.926) radius 36.5016
  circle A36 centre (46.7921, 42.926) radius 34.1821
  circle A37 centre (46.7921, 42.926) radius 29.2524
  circle A38 centre (46.7921, 42.926) radius 27.2128
  circle A39 centre (46.7921, 42.926) radius 21.9649
  circle A40 centre (46.7921, 42.926) radius 19.7247
  circle A41 centre (46.7921, 42.926) radius 14.2135
  line L32 (77.1332, 22.6335) -> (80.9249, 20.4443)
  line L33 (79.5365, 26.7962) -> (83.3282, 24.607)
  line L34 (75.1198, 23.7959) -> (70.8381, 26.2679)
  line L35 (77.5231, 27.9586) -> (73.2415, 30.4306)
  line L36 (71.4687, 31.4541) -> (66.9017, 34.0908)
  line L37 (69.0654, 27.2914) -> (64.4984, 29.9282)
  line L38 (64.9486, 35.2185) -> (60.1258, 38.0029)
  line L39 (62.5453, 31.0558) -> (57.7225, 33.8402)
  circle A42 centre (46.7921, 42.926) radius 40.8714
  circle A43 centre (46.7921, 42.926) radius 36.5016
  circle A44 centre (46.7921, 42.926) radius 34.1821
  circle A45 centre (46.7921, 42.926) radius 29.2524
  circle A46 centre (46.7921, 42.926) radius 27.2128
  circle A47 centre (46.7921, 42.926) radius 21.9649
  circle A48 centre (46.7921, 42.926) radius 19.7247
  circle A49 centre (46.7921, 42.926) radius 14.2135
  line L40 (79.5365, 59.0558) -> (83.3282, 61.245)
  line L41 (77.1332, 63.2185) -> (80.9249, 65.4077)
  line L42 (77.5231, 57.8934) -> (73.2415, 55.4214)
  line L43 (75.1198, 62.0561) -> (70.8381, 59.5841)
  line L44 (69.0654, 58.5606) -> (64.4984, 55.9238)
  line L45 (71.4687, 54.3979) -> (66.9017, 51.7612)
  line L46 (62.5453, 54.7962) -> (57.7225, 52.0118)
  line L47 (64.9486, 50.6335) -> (60.1258, 47.8491)
  circle A50 centre (40.8617, 42.926) radius 1.789
  circle A51 centre (40.8617, 42.926) radius 3.7241
  circle A52 centre (46.7921, 36.9956) radius 1.789
  circle A53 centre (46.7921, 36.9956) radius 3.7241
  circle A54 centre (52.7226, 42.926) radius 1.789
  circle A55 centre (52.7226, 42.926) radius 3.7241
  point P0 (0, 0)
  point P1 (0, 85.852)
  point P2 (60.5711, -19.0602)
  point P3 (-13.7789, 23.8658)
  point P4 (41.6562, 45.8912)
  point P5 (41.6562, 45.8912)
  point P6 (107.3632, 23.8658)
  point P7 (33.0132, -19.0602)
  point P8 (41.6562, 39.9608)
  point P9 (41.6562, 39.9608)
  point P10 (93.5843, 85.852)
  point P11 (93.5843, 0)
  point P12 (33.0132, 104.9122)
  point P13 (107.3632, 61.9862)
  point P14 (51.9281, 39.9608)
  point P15 (51.9281, 39.9608)
  point P16 (-13.7789, 61.9862)
  point P17 (60.5711, 104.9122)
  point P18 (51.9281, 45.8912)
  point P19 (51.9281, 45.8912)
  point P20 (43.8269, 37.7901)
  point P21 (43.8269, 37.7901)
  point P22 (51.9281, 39.9608)
  point P23 (51.9281, 39.9608)
  point P24 (49.7574, 48.0619)
  point P25 (49.7574, 48.0619)
  dimension "d437" = 360
  dimension "d441" = 360
  constraints: 96 end point, 96 point on circle, 56 centre point, 56 coincident, 6 parallel, 1 collinear, 288 other
extrude "Extrusion6" cut sketch "Sketch8" against normal blind 25.4 contours A0 L33 A1 L40 | L41 A1 L0 A0 | A0 L25 A1 L32 | L1 A1 L8 A0 | A0 L17 A1 L24 | L9 A1 L16 A0 | A2 L35 A3 L42 | L43 A3 L2 A2 | A2 L27 A3 L34 | L3 A3 L10 A2 | A2 L19 A3 L26 | L11 A3 L18 A2 | A4 L36 A5 L45 | L44 A5 L5 A4 | A4 L28 A5 L37 | L4 A5 L13 A4 | A4 L20 A5 L29 | L12 A5 L21 A4 | A6 L38 A7 L47 | L46 A7 L7 A6 | A6 L30 A7 L39 | L6 A7 L15 A6 | A6 L22 A7 L31 | L14 A7 L23 A6 | A8 | A9 | A50 | A51 | A52 | A53 | A54 | A55
sketch "Sketch9" plane through (0, 0, 150.495) normal (1, 0, 0) x (0, 0, -1)
  circle A0 centre (13.2643, 75.3758) radius 8.7615
  circle A1 centre (13.2643, 75.3758) radius 6.6331
  constraints: 2 centre point, 1 coincident
extrude "Extrusion7" add sketch "Sketch9" along normal blind 1.27
sketch "Sketch10" plane through (0, 75.3758, 137.2307) normal (1, 0, 0) x (0, 0, -1)
  circle A0 centre (0, 0) radius 6.6331 projected
  point P0 (137.2307, -75.3758)
extrude "Extrusion8" cut sketch "Sketch10" against normal blind 25.4
sketch "Sketch11" plane through (-141.224, 0, 0) normal (-1, 0, 0) x (0, 0, 1)
  line L0 (110.4433, 17.5927) -> (135.8433, 17.5927)
  line L1 (135.8433, 17.5927) -> (135.8433, 4.8927)
  line L2 (135.8433, 4.8927) -> (110.4433, 4.8927)
  line L3 (110.4433, 4.8927) -> (110.4433, 17.5927)
  arc A0 (105.0952, 14.1691) -> (105.0952, 8.3163) centre (106.9686, 11.2427) ccw
  arc A1 (141.153, 8.3755) -> (141.153, 14.1099) centre (139.2723, 11.2427) ccw
  line L4 (110.4433, 17.5927) -> (105.0952, 14.1691)
  line L5 (110.4433, 4.8927) -> (105.0952, 8.3163)
  line L6 (135.8433, 4.8927) -> (141.153, 8.3755)
  line L7 (135.8433, 17.5927) -> (139.2723, 14.6717)
  line L8 (135.8433, 17.5927) -> (141.153, 14.1099)
  dimension "d449" = 25.4
  dimension "d450" = 12.7
  dimension "d451" = 6.858
  constraints: 18 end point, 5 tangent, 4 point on circle, 2 centre point, 2 parallel, 1 horizontal, 1 perpendicular
  measures "d449" distance of L1.end L2.end
  measures "d450" distance of L0.end L1.end
  measures "d451" diameter of A1
extrude "Extrusion9" add sketch "Sketch11" along normal blind 2.54
body "Solid1"
